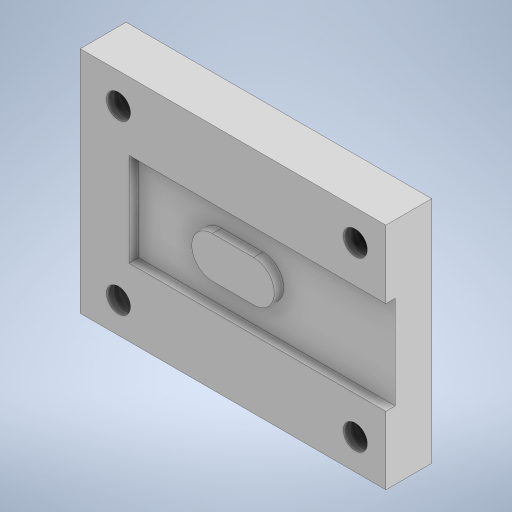
# Autodesk Inventor part: cutter_holder
Saved by Autodesk Inventor 2024.3 (Build 283343000, 343)
## iProperties
Created: 2025-06-10
Part Number: cutter_holder
Material: 一般
Document SubType Name: Modeling
Designer: hikou
Density: 1 g/cm^3
Appearance: 既定
Author: hikou
Autodesk Inventor part; units mm, degrees
ref_plane "YZ Plane" through (0, 0, 0) normal (1, 0, 0) x (0, 1, 0)
ref_plane "XZ Plane" through (0, 0, 0) normal (0, 1, 0) x (-1, 0, 0)
ref_plane "XY Plane" through (0, 0, 0) normal (0, 0, 1) x (1, 0, 0)
sketch "スケッチ1" plane through (0, 0, 0) normal (0, 0, 1) x (1, 0, 0)
  line L0 (-10, -7.5) -> (10, -7.5)
  line L1 (10, -7.5) -> (10, 7.5)
  line L2 (10, 7.5) -> (-10, 7.5)
  line L3 (-10, 7.5) -> (-10, -7.5)
  line L4 (-10, -7.5) -> (10, 7.5) construction
  line L5 (10, -7.5) -> (-10, 7.5) construction
  point P0 (0, 0)
  dimension "d0" = 20
  dimension "d1" = 15
  constraints: 12 end point, 2 midpoint, 2 parallel, 1 horizontal, 1 perpendicular
  measures "d0" distance of L1.end L2.end
  measures "d1" distance of L0.end L1.end
extrude "押し出し1" add sketch "スケッチ1" along normal mid plane 3
sketch "スケッチ2" plane through (0, 0, 1.5) normal (0, 0, 1) x (1, 0, 0)
  line L0 (10, -7.5) -> (10, 7.5) projected
  line L1 (-10, -3.05) -> (10, -3.05)
  line L2 (10, -3.05) -> (10, 3.05)
  line L3 (10, 3.05) -> (-10, 3.05)
  line L4 (-10, 3.05) -> (-10, -3.05)
  line L5 (-10, -3.05) -> (10, 3.05) construction
  line L6 (10, -3.05) -> (-10, 3.05) construction
  point P0 (0, 0)
  dimension "d4" = 6.1
  constraints: 12 end point, 2 midpoint, 2 parallel, 1 horizontal, 1 perpendicular, 1 point on line
  measures "d4" distance between parallel lines of L1 L3
extrude "押し出し2" cut sketch "スケッチ2" against normal blind 0.6
sketch "スケッチ3" plane through (0, 0, 0.9) normal (0, 0, 1) x (1, 0, 0)
  line L0 (-1.35, 0) -> (1.35, 0) construction
  line L1 (-1.35, -1.35) -> (1.35, -1.35)
  line L2 (1.35, 1.35) -> (-1.35, 1.35)
  arc A0 (-1.35, 1.35) -> (-1.35, -1.35) centre (-1.35, 0) ccw
  arc A1 (1.35, -1.35) -> (1.35, 1.35) centre (1.35, 0) ccw
  point P0 (0, 0)
  point P1 (2.7, 0)
  point P2 (-2.7, 0)
  dimension "d7" = 2.7
  dimension "d8" = 5.4
  constraints: 8 end point, 6 point on circle, 4 tangent, 2 centre point, 1 horizontal, 1 midpoint, 1 parallel
  measures "d7" distance between parallel lines of L1 L2
  measures "d8" distance of point (2.7, 0) point (-2.7, 0)
extrude "押し出し3" add sketch "スケッチ3" along normal blind 0.6
sketch "スケッチ4" plane through (0, 0, 0.9) normal (0, 0, 1) x (1, 0, 0)
  line L0 (1.35, -1.35) -> (-1.35, -1.35) projected
  arc A0 (-1.35, 1.35) -> (-1.35, -1.35) centre (-1.35, 0) ccw projected
  line L1 (-1.35, 1.35) -> (1.35, 1.35) projected
  arc A1 (1.35, -1.35) -> (1.35, 1.35) centre (1.35, 0) ccw projected
  line L2 (10, -3.05) -> (-10, -3.05) projected
  line L3 (10, 3.05) -> (10, -3.05) projected
  line L4 (-10, 3.05) -> (10, 3.05) projected
  line L5 (-10, -3.05) -> (-10, 3.05) projected
  line L6 (-10, 3.05) -> (10, 3.05) projected
  line L7 (-6.8, 3.05) -> (-6.8, -3.05)
  arc A2 (-1.35, 1.35) -> (-1.35, -1.35) centre (-1.35, 0) ccw projected
  point P0 (0, 0)
  point P1 (-2.7, 0)
  dimension "d11" = 4.1
  constraints: 2 end point, 2 point on line, 1 perpendicular, 1 point on circle
  measures "d11" distance from line of L7 point (-2.7, 0)
extrude "押し出し4" add sketch "スケッチ4" along normal blind 0.6 contours L2 L5 L4 L7
sketch "スケッチ5" plane through (0, 0, 1.5) normal (0, 0, 1) x (1, 0, 0)
  line L0 (0, 0) -> (2.6024, 0)
  point P0 (-7.5, 5.5)
  point P1 (8, 5.5)
  point P2 (-7.5, -5.5)
  point P3 (8, -5.5)
  dimension "d14" = 5.5
  dimension "d15" = 5.5
  dimension "d16" = 8
  dimension "d17" = 7.5
  constraints: 2 end point, 2 symmetric about line, 1 horizontal
  measures "d14" vertical distance of point (8, 5.5) L0.start
  measures "d15" vertical distance of L0.start point (-7.5, 5.5)
  measures "d16" horizontal distance of point (8, 5.5) L0.start
  measures "d17" horizontal distance of point (-7.5, 5.5) L0.start
hole "穴1" at (-7.5, 5.5, 1.5) at (8, 5.5, 1.5) at (-7.5, -5.5, 1.5) at (8, -5.5, 1.5) direction (0, 0, -1) diameter 1.567 end through all thread size "M2x0.4" class "6H" standard "ISO Metric profile"
equation "\"d15\" = d14"
